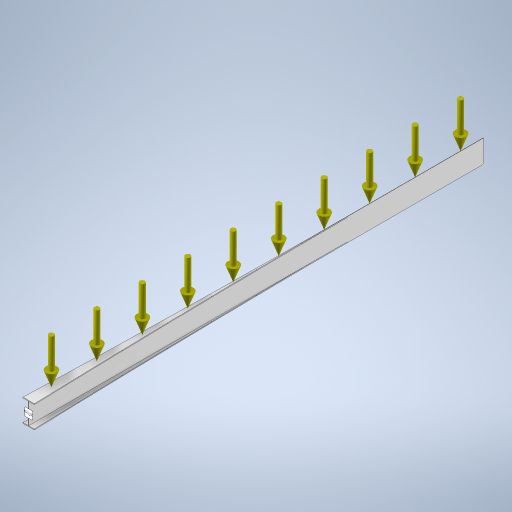
# Autodesk Inventor part: Part2
Saved by Autodesk Inventor 2024 (Build 280153000, 153)
## iProperties
Created: 2024-04-24
Part Number: Part2
Material: Aluminum 2014-T6
Document SubType Name: Modeling
Designer: AcerLaptopOwner
Mass: 8679.45 g
Surface Area: 20167 cm^2
Volume: 3111.73 cm^3
Density: 2.78927 g/cm^3
Appearance: Satin
Author: AcerLaptopOwner
Autodesk Inventor part; units mm, degrees
ref_plane "YZ Plane" through (0, 0, 0) normal (1, 0, 0) x (0, 1, 0)
ref_plane "XZ Plane" through (0, 0, 0) normal (0, 1, 0) x (-1, 0, 0)
ref_plane "XY Plane" through (0, 0, 0) normal (0, 0, 1) x (1, 0, 0)
sketch "Sketch1" plane through (0, 0, 0) normal (0, 1, 0) x (-1, 0, 0)
  point P0 (0, 0)
sketch "Sketch2" plane through (0, 0, 0) normal (0, 0, 1) x (1, 0, 0)
  line L0 (-50, 200) -> (50, 200)
  line L1 (50, 200) -> (50, 0)
  line L2 (50, 0) -> (-50, 0)
  line L3 (-50, 0) -> (-50, 200)
  line L4 (-50, 192.411) -> (-1, 192.411)
  line L5 (-1, 192.411) -> (-1, 7.589)
  line L6 (-1, 7.589) -> (-50, 7.589)
  line L7 (-50, 7.589) -> (-50, 192.411)
  line L8 (50, 192.411) -> (1, 192.411)
  line L9 (1, 192.411) -> (1, 7.589)
  line L10 (1, 7.589) -> (50, 7.589)
  line L11 (50, 7.589) -> (50, 192.411)
  point P0 (0, 0)
  point P1 (0, 0)
  dimension "d0" = 100
  dimension "d1" = 2
  dimension "d2" = 7.589
  dimension "d3" = 7.589
  dimension "d4" = 200
  constraints: 24 end point, 6 parallel, 4 point on line, 3 horizontal, 3 perpendicular, 1 coincident, 1 collinear, 1 midpoint
  measures "d0" distance of L0.start L0.end
  measures "d1" distance between parallel lines of L9 L5
  measures "d2" distance between parallel lines of L4 L0
  measures "d3" distance between parallel lines of L2 L6
  measures "d4" distance of L0.end L1.end
extrude "Extrusion1" add sketch "Sketch2" along normal blind 4000 contours L0 L1 L8 L9 L10 L2 L3 L6 L5 L4
sketch "Sketch5" plane through (-50, 200, 0) normal (0, 1, 0) x (1, 0, 0)
  line L0 (100, -3600) -> (100, -3200)
  line L1 (100, 0) -> (100, -4000) projected
  line L2 (100, 0) -> (100, -4000) projected
  line L3 (100, -4000) -> (100, -3600)
  line L4 (100, -4000) -> (0, -4000) projected
  line L5 (100, -3600) -> (100, -3200)
  line L6 (100, -3200) -> (100, -2800)
  line L7 (69.25, -2800) -> (77.9, -3200)
  line L8 (100, -2800) -> (100, -2400)
  line L9 (62.1, -2400) -> (69.25, -2800)
  line L10 (88.15, -3600) -> (100, -4000)
  line L11 (77.9, -3200) -> (88.15, -3600)
  line L12 (100, -2400) -> (100, -2000)
  line L13 (100, -2000) -> (100, -1600)
  line L14 (56.45, -2000) -> (62.1, -2400)
  line L15 (52.15, -1600) -> (56.45, -2000)
  line L16 (100, -1600) -> (100, -1200)
  line L17 (100, -1200) -> (100, -800)
  line L18 (100, -800) -> (100, -400)
  line L19 (100, -400) -> (100, 0)
  line L20 (100, 0) -> (0, 0) projected
  line L21 (49, 0) -> (49, -4000) projected
  line L22 (51, -1200) -> (52.15, -1600)
  line L23 (51, -800) -> (51, -1200)
  line L24 (51, -400) -> (51, -800)
  line L25 (100, 0) -> (51, 0)
  line L26 (51, -400) -> (51, 0)
  point P0 (50, 0)
  dimension "d23" = 400
  dimension "d25" = 400
  dimension "d27" = 400
  dimension "d28" = 30.75
  dimension "d29" = 400
  dimension "d30" = 37.9
  dimension "d31" = 11.85
  dimension "d32" = 22.1
  dimension "d33" = 400
  dimension "d34" = 400
  dimension "d35" = 43.55
  dimension "d37" = 400
  dimension "d38" = 400
  dimension "d39" = 400
  dimension "d40" = 400
  dimension "d43" = 47.85
  dimension "d44" = 49
  dimension "d45" = 49
  dimension "d46" = 49
  dimension "d47" = 49
  constraints: 44 end point, 3 collinear, 2 point on line, 1 vertical, 8 other
  measures "d23" distance of L1.end L0.start
  measures "d25" distance of L0.start L0.end
  measures "d27" distance of L0.end L6.end
  measures "d28" distance of L6.end L7.start
  measures "d29" distance of L6.end L8.end
  measures "d30" distance of L8.end L9.start
  measures "d31" distance of L0.start L10.start
  measures "d32" distance of L0.end L7.end
  measures "d33" distance of L8.end L12.end
  measures "d34" distance of L12.end L13.end
  measures "d35" distance of L12.end L14.start
  measures "d37" distance of L13.end L16.end
  measures "d38" distance of L16.end L17.end
  measures "d39" distance of L17.end L18.end
  measures "d40" distance of L18.end L1.start
  measures "d43" distance of L15.start L13.end
  measures "d44" distance of L16.end L22.start
  measures "d45" distance of L17.end L23.start
  measures "d46" distance of L18.end L24.start
  measures "d47" distance of L1.start L25.end
extrude "Extrusion4" cut sketch "Sketch5" against normal blind 1000 contours L1 L10 L11 L7 L9 L14 L15 L22 L23 L24 L26 L20 L0
split "Split1" plane through (0, 0, 0) removes the side toward (-1, 0, 0)
mirror "Mirror1" about plane through (0, 0, 0) normal (1, 0, 0)
sketch "Sketch6" plane through (1, 200, 1200) normal (0, 1, 0) x (1, 0, 0)
  line L0 (-51, -2800) -> (49, -2800) projected
  line L1 (-51, -2800) -> (-1, -2800)
  line L2 (-1, -2800) -> (-1, -2600)
  circle A0 centre (-1, -2600) radius 0.5
  point P0 (-1, 1200)
  dimension "d50" = 200
  dimension "d51" = 1
  constraints: 4 end point, 1 centre point, 1 coincident, 1 midpoint, 1 vertical
  measures "d50" distance of L1.end L2.end
  measures "d51" diameter of A0
extrude "Extrusion5" add sketch "Sketch6" along normal blind 0.001
pattern_linear "Rectangular Pattern1" count 10 spacing 400 along (0, 0, -1) of "Extrusion5"
equation "\"d3\" = d2"
body "Solid1"
